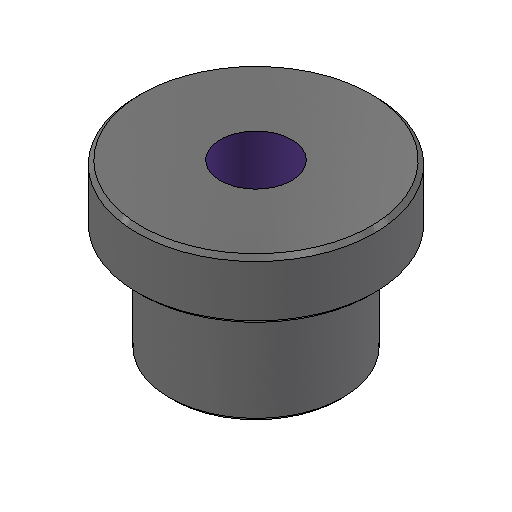
# Autodesk Inventor part: TL20240701-10110CV-012
Saved by Autodesk Inventor 2022.5 (Build 265521000, 521)
## iProperties
Category: DRIVE UNIT ASSY
Manager: 호상태
Company: 현대 트랜시스(대유)
Created: 2023-01-25
Part Number: TL20240701-10110CV-012
Checked By: 김형민
Engr Approved By: 김시현
User Status: 1 x18
Material: S45C
Description: 0
Document SubType Name: Modeling
Mfg Approved By: 호상태
Designer: 박성규
Stock Number: 012
Density: 7.87 g/cm^3
Appearance: Plating Zinc White
Project: SW PJT
DETAIL: Coveryor Assembly
M/C TITLE: MEa/NEa차종 시트조립라인
SPECIFICATION: TL20221201-000000CV-050
DocNumber: 221118_Standard_v1
Folder: .\
VDS_Category: 엔지니어링
Detail Description: Processed products
Title: BAR
Subject: SW차종 시트조립라인
Author: 박성규
Revision Number: A
Autodesk Inventor part; units mm, degrees
ref_plane "YZ Plane" through (0, 0, 0) normal (1, 0, 0) x (0, 1, 0)
ref_plane "XZ Plane" through (0, 0, 0) normal (0, 1, 0) x (-1, 0, 0)
ref_plane "XY Plane" through (0, 0, 0) normal (0, 0, 1) x (1, 0, 0)
sketch "스케치8" plane through (0, 0, 0) normal (0, 1, 0) x (-1, 0, 0)
  circle A0 centre (0, 0) radius 30
  dimension "d38" = 60
  constraints: 1 centre point, 1 coincident
  measures "d38" diameter of A0
extrude "돌출3" add sketch "스케치8" along normal blind 15
sketch "스케치10" plane through (0, 0, 0) normal (0, -1, 0) x (1, 0, 0)
  circle A0 centre (0, 0) radius 30 construction
  circle A1 centre (0, 0) radius 22
  dimension "d51" = 44
  constraints: 1 centre point, 1 coincident
  measures "d51" diameter of A1
extrude "돌출4" add sketch "스케치10" along normal blind 27
sketch "스케치11" plane through (0, 15, 0) normal (0, 1, 0) x (1, 0, 0)
  circle A0 centre (0, 0) radius 30 construction
  constraints: 1 coincident
hole "구멍4" at (0, 15, 0) direction (0, -1, 0) diameter 11 end through all counterbore diameter 18 counterbore depth 16 clearance for "Socket Head Cap Screw ISO 4762" size "M10" standard "ISO"
chamfer "모따기2" distance 1 angle 45 3 edges at (30, 15, 0) (30, 0, 0) (-22, -27, 0)
